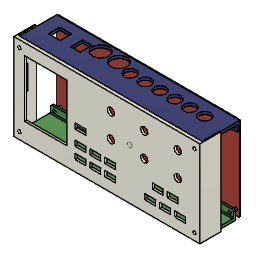
pfm3EnclosureV2 (Autodesk Fusion 360 design; units mm, degrees)
Autodesk Fusion 360 part; units mm, degrees
sketch "Top face" plane through (0, 0, 0) normal (0, 0, 1) x (1, 0, 0)
  circle A0 centre (6.01, 7.71) radius 1.85
  circle A1 centre (200.32, 7.71) radius 1.75
  line L0 (11.86, 83.56) -> (58.86, 83.56)
  line L1 (58.86, 83.56) -> (58.86, 20.56)
  line L2 (58.86, 20.56) -> (11.86, 20.56)
  line L3 (11.86, 20.56) -> (11.86, 83.56)
  circle A2 centre (107.61, 77.687) radius 4
  circle A3 centre (144.694, 77.687) radius 4
  circle A4 centre (181.778, 77.687) radius 4
  circle A5 centre (107.61, 51.017) radius 4
  circle A6 centre (144.694, 51.017) radius 4
  circle A7 centre (181.778, 51.017) radius 4
  line L4 (79.828, 11.822) -> (67.828, 11.822)
  line L5 (67.828, 11.822) -> (67.828, 17.822)
  line L6 (67.828, 17.822) -> (79.828, 17.822)
  line L7 (79.828, 17.822) -> (79.828, 11.822)
  line L8 (79.828, 11.822) -> (67.828, 17.822) construction
  line L9 (67.828, 11.822) -> (79.828, 17.822) construction
  line L10 (84.338, 17.822) -> (96.338, 17.822)
  line L11 (84.338, 11.822) -> (84.338, 17.822)
  line L12 (96.338, 11.822) -> (84.338, 11.822)
  line L13 (96.338, 17.822) -> (96.338, 11.822)
  line L14 (100.848, 17.822) -> (112.848, 17.822)
  line L15 (100.848, 11.822) -> (100.848, 17.822)
  line L16 (112.848, 11.822) -> (100.848, 11.822)
  line L17 (112.848, 17.822) -> (112.848, 11.822)
  line L18 (67.828, 30.522) -> (79.828, 30.522)
  line L19 (67.828, 24.522) -> (67.828, 30.522)
  line L20 (79.828, 24.522) -> (67.828, 24.522)
  line L21 (79.828, 30.522) -> (79.828, 24.522)
  line L22 (84.338, 30.522) -> (96.338, 30.522)
  line L23 (84.338, 24.522) -> (84.338, 30.522)
  line L24 (96.338, 24.522) -> (84.338, 24.522)
  line L25 (96.338, 30.522) -> (96.338, 24.522)
  line L26 (100.848, 30.522) -> (112.848, 30.522)
  line L27 (100.848, 24.522) -> (100.848, 30.522)
  line L28 (112.848, 24.522) -> (100.848, 24.522)
  line L29 (112.848, 30.522) -> (112.848, 24.522)
  line L30 (79.828, 41.032) -> (67.828, 41.032)
  line L31 (67.828, 41.032) -> (67.828, 47.032)
  line L32 (67.828, 47.032) -> (79.828, 47.032)
  line L33 (79.828, 47.032) -> (79.828, 41.032)
  line L34 (79.828, 41.032) -> (67.828, 47.032) construction
  line L35 (67.828, 41.032) -> (79.828, 47.032) construction
  line L36 (157.298, 11.822) -> (145.298, 11.822)
  line L37 (145.298, 11.822) -> (145.298, 17.822)
  line L38 (145.298, 17.822) -> (157.298, 17.822)
  line L39 (157.298, 17.822) -> (157.298, 11.822)
  line L40 (157.298, 11.822) -> (145.298, 17.822) construction
  line L41 (145.298, 11.822) -> (157.298, 17.822) construction
  line L42 (173.808, 11.822) -> (161.808, 11.822)
  line L43 (173.808, 17.822) -> (173.808, 11.822)
  line L44 (161.808, 11.822) -> (161.808, 17.822)
  line L45 (161.808, 17.822) -> (173.808, 17.822)
  line L46 (190.318, 11.822) -> (178.318, 11.822)
  line L47 (190.318, 17.822) -> (190.318, 11.822)
  line L48 (178.318, 11.822) -> (178.318, 17.822)
  line L49 (178.318, 17.822) -> (190.318, 17.822)
  line L50 (165.553, 26.3) -> (153.553, 26.3)
  line L51 (153.553, 26.3) -> (153.553, 32.3)
  line L52 (153.553, 32.3) -> (165.553, 32.3)
  line L53 (165.553, 32.3) -> (165.553, 26.3)
  line L54 (165.553, 26.3) -> (153.553, 32.3) construction
  line L55 (153.553, 26.3) -> (165.553, 32.3) construction
  line L56 (182.063, 26.3) -> (170.063, 26.3)
  line L57 (170.063, 26.3) -> (170.063, 32.3)
  line L58 (170.063, 32.3) -> (182.063, 32.3)
  line L59 (182.063, 32.3) -> (182.063, 26.3)
  circle A8 centre (128.435, 55.843) radius 2.5
  line L60 (-5.2146, 48.0325) -> (227.1425, 48.0325) construction
  line L61 (106.155, 103.4224) -> (106.155, -13.7368) construction
  circle A9 centre (6.01, 88.355) radius 1.85
  circle A10 centre (200.32, 88.355) radius 1.75
  line L62 (0, 0) -> (206.33, 0)
  line L63 (206.33, 0) -> (206.33, 96.065)
  line L64 (206.33, 96.065) -> (0, 96.065)
  line L65 (0, 96.065) -> (0, 0)
  line L66 (205.12, 96.065) -> (205.12, 0)
  line L67 (1.21, 96.065) -> (1.21, 0)
  line L68 (1.21, 91.455) -> (2.01, 91.455)
  line L69 (2.01, 91.455) -> (2.01, 4.61)
  line L70 (2.01, 4.61) -> (1.21, 4.61)
  line L71 (1.21, 4.61) -> (1.21, 91.455)
  line L72 (205.12, 91.455) -> (204.32, 91.455)
  line L73 (204.32, 91.455) -> (204.32, 4.61)
  line L74 (204.32, 4.61) -> (205.12, 4.61)
  line L75 (205.12, 4.61) -> (205.12, 91.455)
  line L76 (1.21, 94.855) -> (211.1, 94.855)
  line L77 (1.21, 1.21) -> (205.12, 1.21)
  point P0 (6.01, 7.71)
  point P1 (63.795, 7.71)
  point P2 (73.828, 14.822)
  point P3 (73.828, 44.032)
  point P4 (151.298, 14.822)
  point P5 (159.553, 29.3)
  point P6 (128.435, 55.843)
  dimension "d3" = 3.7
  dimension "d11" = 3.5
  dimension "d12" = 194.31
  dimension "d15" = 57.785
  dimension "d16" = 63
  dimension "d17" = 47
  dimension "d20" = 8
  dimension "d23" = 37.084
  dimension "d24" = -26.67
  dimension "d25" = 12
  dimension "d26" = 6
  dimension "d27" = 7.112
  dimension "d28" = 10.033
  dimension "d31" = 16.51
  dimension "d32" = 12.7
  dimension "d34" = 43.815
  dimension "d35" = 69.977
  dimension "d36" = 12
  dimension "d37" = 6
  dimension "d38" = 10.033
  dimension "d39" = 36.322
  dimension "d40" = 12
  dimension "d41" = 6
  dimension "d42" = 7.112
  dimension "d45" = 16.51
  dimension "d46" = 0
  dimension "d47" = 12
  dimension "d48" = 6
  dimension "d51" = 16.51
  dimension "d52" = 0
  dimension "d53" = 21.59
  dimension "d54" = 95.758
  dimension "d60" = 16.51
  dimension "d61" = 16.51
  dimension "d62" = 12.7
  dimension "d63" = 16.51
  dimension "d64" = 16.51
  dimension "d65" = 87.503
  dimension "d69" = 48.133
  dimension "d70" = 64.64
  dimension "d85" = 37.084
  dimension "d86" = 37.084
  dimension "d87" = 26.67
  dimension "d89" = 5
  dimension "d92" = 5.85
  dimension "d93" = 12.85
  dimension "d275" = 80.645
  dimension "d281" = 1.21
  dimension "d282" = 1.21
  dimension "d283" = 0.8
  dimension "d284" = 0.8
  dimension "d285" = 1.21
  dimension "d286" = 1.21
  dimension "d294" = 3.4
  dimension "d295" = 3.4
  dimension "d296" = 3.4
  dimension "d297" = 3.4
  dimension "d315" = 6.5
  dimension "d316" = 6.5
  dimension "d319" = 4
  dimension "d320" = 4
  constraint horizontal P0 P1
  constraint horizontal L0
  constraint vertical L1
  constraint horizontal L2
  constraint vertical L3
  constraint horizontal L4
  constraint perpendicular L4 L5
  constraint parallel L4 L6
  constraint parallel L5 L7
  constraint coincident L8 P2
  constraint coincident L9 P2
  constraint horizontal L30
  constraint perpendicular L30 L31
  constraint parallel L30 L32
  constraint parallel L31 L33
  constraint coincident L34 P3
  constraint coincident L35 P3
  constraint horizontal L36
  constraint perpendicular L36 L37
  constraint parallel L36 L38
  constraint parallel L37 L39
  constraint coincident L40 P4
  constraint coincident L41 P4
  constraint horizontal L50
  constraint perpendicular L50 L51
  constraint parallel L50 L52
  constraint parallel L51 L53
  constraint coincident L54 P5
  constraint coincident L55 P5
  constraint coincident P6 A8.centre
  constraint coincident P0 A0.centre
  constraint horizontal L60
  constraint symmetric A0 L60 A9
  constraint symmetric A1 L60 A10
  constraint horizontal P0 A1.centre
  constraint horizontal L62
  constraint vertical L63
  constraint horizontal L64
  constraint vertical L65
  constraint coincident L62.start L65.end
  constraint coincident L64 L66.start
  constraint coincident L62 L66.end
  constraint perpendicular L62 L66
  constraint coincident L64 L67.start
  constraint coincident L62 L67.end
  constraint perpendicular L62 L67
  constraint horizontal L68
  constraint vertical L69
  constraint horizontal L70
  constraint vertical L71
  constraint coincident L67 L68.start
  constraint horizontal L72
  constraint vertical L73
  constraint horizontal L74
  constraint vertical L75
  constraint coincident L66 L72.start
  constraint horizontal L76
  constraint coincident L67 L76.start
  constraint horizontal L77
  constraint coincident L67 L77.start
  constraint coincident L66 L77.end
  measures "d3" diameter of A0
  measures "d11" diameter of A1
  measures "d12" distance of P0 A1.centre
  measures "d15" horizontal distance of P0 P1
  measures "d16" distance of L0.start L2.end
  measures "d17" distance of L0.start L0.end
  measures "d20" diameter of A2
  measures "d25" distance of L5.end L6.end
  measures "d26" distance of L4.end L5.end
  measures "d27" vertical distance of P1 P2
  measures "d28" horizontal distance of P1 P2
  measures "d34" horizontal distance of P1 A2.centre
  measures "d35" vertical distance of P1 A2.centre
  measures "d36" distance of L31.end L32.end
  measures "d37" distance of L30.end L31.end
  measures "d38" horizontal distance of P1 P3
  measures "d39" vertical distance of P1 P3
  measures "d40" distance of L37.end L38.end
  measures "d41" distance of L36.end L37.end
  measures "d42" vertical distance of P1 P4
  measures "d47" distance of L51.end L52.end
  measures "d48" distance of L50.end L51.end
  measures "d53" vertical distance of P1 P5
  measures "d54" horizontal distance of P1 P5
  measures "d60" distance of L19 L23
  measures "d61" distance of L23 L27
  measures "d62" distance of L16 L28
  measures "d63" distance of L37 L44
  measures "d64" distance of L44 L48
  measures "d65" horizontal distance of P1 P4
  measures "d69" vertical distance of P1 P6
  measures "d70" horizontal distance of P1 P6
  measures "d85" distance of A3.centre A4.centre
  measures "d86" distance of A2.centre A3.centre
  measures "d87" distance of A2.centre A5.centre
  measures "d89" diameter of A8
  measures "d92" distance of P0 L3
  measures "d93" distance of P0 L2
  measures "d275" distance of P0 A9.centre
  measures "d281" distance of L63 L66
  measures "d282" distance of L65 L67
  measures "d283" distance of L69 L71
  measures "d284" distance of L72.start L72.end
  measures "d285" distance of L64 L76
  measures "d286" distance of L66.end L77
  measures "d294" distance of L68 L76
  measures "d295" distance of L70 L77
  measures "d296" distance of L74 L77
  measures "d297" distance of L72 L76
  measures "d315" distance of A9.centre L76
  measures "d316" distance of P0 L77
  measures "d319" distance of A1.centre L73
  measures "d320" distance of P0 L69
extrude "Extrude27" add sketch "Top face" against normal blind 1.2 contours L62 L66 L67 L77 | L64 L66 L67 L76 makes body 1 at (69.18, 95.6617, 0) makes body 2 at (69.18, 0.8067, 0)
extrude "Extrude26" add sketch "Top face" along normal blind 2.4 contours A8 | L62 L64 L65 L67 L71 | L62 L66 L67 L77 | L62 L63 L66 L75 L76 | L66 L67 L68 L69 L70 L72 L73 L74 L76 L77 | L64 L66 L67 L76 | L67 L68 L69 L70 L71 | L63 L64 L66 L76 | L66 L72 L73 L74 L75 bodies 1 2
extrude "Extrude31" cut sketch "Top face" along normal blind 1.8 contours A8 bodies 1
extrude "Extrude28" add sketch "Top face" against normal blind 21 contours L62 L64 L65 L67 L71 | L62 L63 L66 L75 L76 | L67 L68 L69 L70 L71 | L63 L64 L66 L76 | L66 L72 L73 L74 L75 bodies 1
ref_plane "WorkPlane3" through (103.165, 94.855, -0.6) normal (0, -1, 0) x (-1, 0, 0)
sketch "Back face" plane through (0, 94.855, 0) normal (0, -1, 0) x (-1, 0, 0)
  line L0 (20.1532, 21.6) -> (-214.6841, 21.6) construction
  circle A0 centre (-181.27, 28.1) radius 6.5
  circle A1 centre (-164.76, 28.1) radius 6.5
  circle A2 centre (-148.25, 28.1) radius 6.5
  circle A3 centre (-131.74, 28.1) radius 6.5
  circle A4 centre (-115.23, 28.1) radius 6.5
  circle A5 centre (-98.72, 28.1) radius 6.5
  circle A6 centre (-81.58, 32.6) radius 9
  circle A7 centre (-61.26, 32.6) radius 9
  line L1 (-40.13, 33.6) -> (-50.63, 33.6)
  line L2 (-50.63, 33.6) -> (-50.63, 20.6)
  line L3 (-50.63, 20.6) -> (-40.13, 20.6)
  line L4 (-40.13, 20.6) -> (-40.13, 33.6)
  line L5 (-40.13, 33.6) -> (-50.63, 20.6) construction
  line L6 (-50.63, 33.6) -> (-40.13, 20.6) construction
  line L7 (-15.37, 20.6) -> (-28.41, 20.6)
  line L8 (-28.41, 20.6) -> (-28.41, 33.2)
  line L9 (-28.41, 33.2) -> (-15.37, 33.2)
  line L10 (-15.37, 33.2) -> (-15.37, 20.6)
  line L11 (-15.37, 20.6) -> (-28.41, 33.2) construction
  line L12 (-28.41, 20.6) -> (-15.37, 33.2) construction
  line L13 (-1.61, 43.6) -> (-204.72, 43.6)
  line L14 (-204.72, 43.6) -> (-204.72, 0.3)
  line L15 (-204.72, 0.3) -> (-1.61, 0.3)
  line L16 (-1.61, 0.3) -> (-1.61, 43.6)
  line L17 (-206.33, 0) -> (0, 0)
  line L18 (-1.21, 1.2) -> (-1.21, 21)
  line L19 (-205.12, 1.2) -> (-205.12, 21)
  line L20 (-200.32, 1.2) -> (-200.32, -3.6)
  point P0 (-45.38, 27.1)
  point P1 (-21.89, 26.9)
  dimension "d110" = 13
  dimension "d115" = 16.51
  dimension "d116" = 0
  dimension "d118" = 18
  dimension "d122" = 20.32
  dimension "d123" = 0
  dimension "d124" = 16.51
  dimension "d125" = 20.32
  dimension "d126" = 10.5
  dimension "d127" = 13
  dimension "d130" = 13.04
  dimension "d131" = 12.6
  dimension "d298" = 21.6
  dimension "d299" = 0.3
  dimension "d300" = 43.6
  dimension "d301" = 6.5
  dimension "d302" = 11
  dimension "d303" = 1
  dimension "d304" = 1
  dimension "d305" = 0.4
  dimension "d306" = 0.4
  dimension "d344" = 19.05
  dimension "d351" = 118.74
  dimension "d352" = 154.94
  dimension "d353" = 178.43
  dimension "d354" = 22
  constraint horizontal L1
  constraint perpendicular L1 L2
  constraint parallel L1 L3
  constraint parallel L2 L4
  constraint coincident L5 P0
  constraint coincident L6 P0
  constraint horizontal L7
  constraint perpendicular L7 L8
  constraint parallel L7 L9
  constraint parallel L8 L10
  constraint coincident L11 P1
  constraint coincident L12 P1
  constraint horizontal L13
  constraint vertical L14
  constraint horizontal L15
  constraint vertical L16
  measures "d110" diameter of A0
  measures "d118" diameter of A6
  measures "d124" distance of A0.centre A1.centre
  measures "d125" distance of A6.centre A7.centre
  measures "d126" distance of L2.end L3.end
  measures "d127" distance of L1.end L2.end
  measures "d130" distance of L8.end L9.end
  measures "d131" distance of L7.end L8.end
  measures "d298" distance of L0 L17
  measures "d299" distance of L15 L17
  measures "d300" distance of L13 L17
  measures "d301" distance of L0 A0.centre
  measures "d302" distance of L0 A6.centre
  measures "d303" distance of L0 L7
  measures "d304" distance of L0 L3
  measures "d305" distance of L16 L18
  measures "d306" distance of L14 L19
  measures "d344" distance of A0.centre L20
  measures "d351" horizontal distance of A6.centre L20.start
  measures "d352" distance of P0 L20
  measures "d353" distance of P1 L20
  measures "d354" distance of L0 L13
extrude "Extrude29" add sketch "Back face" along normal blind 3 separate body makes body 3
sketch "Bottom hole" plane through (0, 0, -43.6) normal (0, 0, -1) x (-1, 0, 0)
  line L0 (-1.61, 94.855) -> (-204.72, 94.855)
  line L1 (-204.72, 94.855) -> (-204.72, 91.855)
  line L2 (-204.72, 91.855) -> (-1.61, 91.855)
  line L3 (-1.61, 91.855) -> (-1.61, 94.855)
  line L4 (-204.72, 91.855) -> (-184.72, 91.855)
  line L5 (-184.72, 91.855) -> (-184.72, 83.855)
  line L6 (-184.72, 83.855) -> (-204.72, 83.855)
  line L7 (-204.72, 83.855) -> (-204.72, 91.855)
  line L8 (-1.61, 91.855) -> (-21.61, 91.855)
  line L9 (-21.61, 91.855) -> (-21.61, 83.855)
  line L10 (-21.61, 83.855) -> (-1.61, 83.855)
  line L11 (-1.61, 83.855) -> (-1.61, 91.855)
  circle A0 centre (-200.32, 88.355) radius 1.75
  circle A1 centre (-6.01, 88.355) radius 1.85
  dimension "d309" = 20
  dimension "d310" = 8
  dimension "d311" = 20
  dimension "d312" = 8
  constraint horizontal L4
  constraint vertical L5
  constraint horizontal L6
  constraint vertical L7
  constraint coincident L1.end L2.start
  constraint horizontal L8
  constraint vertical L9
  constraint horizontal L10
  constraint vertical L11
  constraint coincident L2.end L3.start
  measures "d309" distance of L1.end L4.end
  measures "d310" distance of L1.end L6.end
  measures "d311" distance of L2.end L8.end
  measures "d312" distance of L2.end L10.end
extrude "Extrude30" add sketch "Bottom hole" against normal blind 2 contours L2 L8 L9 L10 L11 | L2 L4 L5 L6 L7 bodies 3
sketch "OLD SD" plane through (0, 0, 0) normal (-1, 0, 0) x (0, 0, 1)
  line L0 (-0.1, 4.63) -> (-0.1, 92.645)
  line L1 (-5.1, 64.855) -> (-11.1, 64.855)
  line L2 (-11.1, 64.855) -> (-11.1, 37.855)
  line L3 (-11.1, 37.855) -> (-5.1, 37.855)
  line L4 (-5.1, 37.855) -> (-5.1, 64.855)
  line L5 (0, 96.065) -> (0, 0)
  line L6 (-0.3, 91.855) -> (-41.6, 91.855)
  dimension "d232" = 5
  dimension "d233" = 6
  dimension "d235" = 27
  dimension "d327" = 27
  constraint horizontal L1
  constraint vertical L2
  constraint horizontal L3
  constraint vertical L4
  measures "d232" distance of L0 L4
  measures "d233" distance of L2 L4
  measures "d235" distance of L1 L3
  measures "d327" distance of L1 L6
extrude "Extrude32" cut sketch "OLD SD" against normal up to surface (2.01 mm away) bodies 1
sketch "Front" plane through (0, 1.21, 0) normal (0, 1, 0) x (-1, 0, 0)
  line L0 (-1.21, 0) -> (-205.12, 0)
  line L1 (-205.12, 0) -> (-205.12, -1.2)
  line L2 (-205.12, -1.2) -> (-1.21, -1.2)
  line L3 (-1.21, -1.2) -> (-1.21, 0)
  line L4 (-1.61, -38.6) -> (-204.72, -38.6)
  line L5 (-204.72, -38.6) -> (-204.72, -0.4)
  line L6 (-204.72, -0.4) -> (-1.61, -0.4)
  line L7 (-1.61, -0.4) -> (-1.61, -38.6)
  line L8 (-1.21, -1.2) -> (-1.21, -21)
  line L9 (-205.12, -1.2) -> (-205.12, -21)
  line L10 (-206.33, 0) -> (0, 0)
  dimension "d330" = 0.4
  dimension "d331" = 0.4
  dimension "d332" = 0.4
  dimension "d333" = 38.2
  constraint horizontal L4
  constraint vertical L5
  constraint horizontal L6
  constraint vertical L7
  measures "d330" distance of L7 L8
  measures "d331" distance of L5 L9
  measures "d332" distance of L6 L10
  measures "d333" distance of L4 L6
extrude "Extrude33" add sketch "Front" along normal blind 3 separate body contours L2 L4 L5 L7 makes body 4
sketch "Front hole" plane through (0, 0, -38.6) normal (0, 0, -1) x (-1, 0, 0)
  line L0 (-204.72, 1.21) -> (-1.61, 1.21)
  line L1 (-1.61, 1.21) -> (-1.61, 4.21)
  line L2 (-1.61, 4.21) -> (-204.72, 4.21)
  line L3 (-204.72, 4.21) -> (-204.72, 1.21)
  line L4 (-204.72, 4.21) -> (-184.72, 4.21)
  line L5 (-184.72, 4.21) -> (-184.72, 12.21)
  line L6 (-184.72, 12.21) -> (-204.72, 12.21)
  line L7 (-204.72, 12.21) -> (-204.72, 4.21)
  line L8 (-1.61, 4.21) -> (-21.61, 4.21)
  line L9 (-21.61, 4.21) -> (-21.61, 12.21)
  line L10 (-21.61, 12.21) -> (-1.61, 12.21)
  line L11 (-1.61, 12.21) -> (-1.61, 4.21)
  circle A0 centre (-6.01, 7.71) radius 1.85
  circle A1 centre (-200.32, 7.71) radius 1.75
  dimension "d336" = 20
  dimension "d337" = 8
  dimension "d338" = 20
  dimension "d339" = 8
  constraint horizontal L4
  constraint vertical L5
  constraint horizontal L6
  constraint vertical L7
  constraint coincident L2.end L3.start
  constraint horizontal L8
  constraint vertical L9
  constraint horizontal L10
  constraint vertical L11
  constraint coincident L1.end L2.start
  measures "d336" distance of L2.end L4.end
  measures "d337" distance of L2.end L6.end
  measures "d338" distance of L1.end L8.end
  measures "d339" distance of L1.end L10.end
extrude "Extrude34" add sketch "Front hole" against normal blind 2 contours L2 L4 L5 L6 L7 | L2 L8 L9 L10 L11 bodies 4
sketch "bottom" plane through (0, 0, -43.6) normal (0, 0, -1) x (-1, 0, 0)
  circle A0 centre (-6.01, 88.355) radius 1.85
  circle A1 centre (-200.32, 88.355) radius 1.75
  line L0 (-1.61, 94.855) -> (-204.72, 94.855)
  line L1 (-204.72, 94.855) -> (-204.72, 83.855)
  line L2 (-204.72, 83.855) -> (-184.72, 83.855)
  line L3 (-184.72, 83.855) -> (-184.72, 91.855)
  line L4 (-184.72, 91.855) -> (-21.61, 91.855)
  line L5 (-21.61, 91.855) -> (-21.61, 83.855)
  line L6 (-21.61, 83.855) -> (-1.61, 83.855)
  line L7 (-1.61, 83.855) -> (-1.61, 94.855)
  line L8 (-1.61, 94.855) -> (-204.72, 94.855)
  line L9 (-204.72, 94.855) -> (-204.72, 1.21)
  line L10 (-204.72, 1.21) -> (-1.61, 1.21)
  line L11 (-1.61, 1.21) -> (-1.61, 94.855)
  circle A2 centre (-200.32, 88.355) radius 1.75
  circle A3 centre (-6.01, 88.355) radius 1.85
  circle A4 centre (-6.01, 7.71) radius 1.85
  circle A5 centre (-200.32, 7.71) radius 1.75
  point P0 (-204.72, 1.21)
  point P1 (-1.61, 94.855)
  constraint horizontal L8
  constraint vertical L9
  constraint horizontal L10
  constraint vertical L11
  constraint coincident P0 L9.end
  constraint coincident P1 L0.start
extrude "Extrude35" add sketch "Bottom hole" sketch "bottom" along normal blind 0.9 separate body contours L2 L8 L9 L10 L11 of sketch 2 makes body 5
fillet "Fillet6" radius 2 4 edges at (1.61, 83.855, -42.6) (21.61, 83.855, -42.6) (184.72, 83.855, -42.6) (204.72, 83.855, -42.6) on bodies 3
fillet "Fillet7" radius 2 4 edges at (204.72, 12.21, -37.6) (184.72, 12.21, -37.6) (21.61, 12.21, -37.6) (1.61, 12.21, -37.6) on bodies 4
fillet "Fillet8" radius 1.5 4 edges at (1.61, 1.21, -44.05) (1.61, 94.855, -44.05) (204.72, 94.855, -44.05) (204.72, 1.21, -44.05) on bodies 5
fillet "Fillet9" radius 1.5 2 edges at (2.01, 48.0325, 0) (204.32, 48.0325, 0) on bodies 1
fillet "Fillet10" radius 1 2 edges at (11.61, 91.855, -41.6) (194.72, 91.855, -41.6) on bodies 3
fillet "Fillet11" radius 1 2 edges at (194.72, 4.21, -36.6) (11.61, 4.21, -36.6) on bodies 4
equation "d298 = 20 mm + 1.6 mm"
equation "d300 = 20 mm + 20 mm + 1.6 mm + 2 mm"
equation "d333 = 15 mm + 20 mm + 1.6 mm + 2 mm - 0.4 mm"
named bodies: "Top", "Rear", "front", "bottom"
